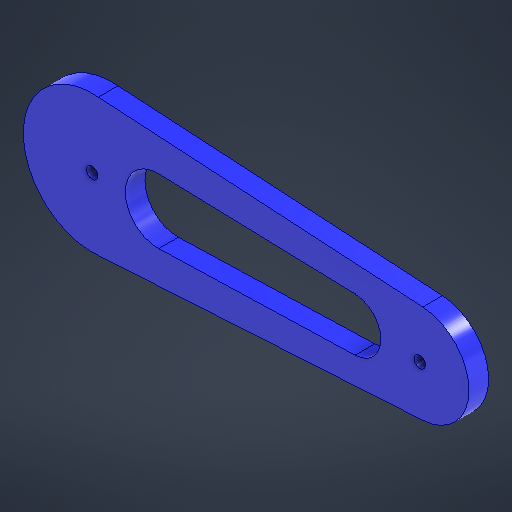
# Autodesk Inventor part: Tibia
Saved by Autodesk Inventor 2026.2 (Build 302298010, 298A)
## iProperties
Created: 2026-07-24
Part Number: Tibia
Material: Generic
Document SubType Name: Modeling
Designer: Entity
Mass: 19.7765 g
Surface Area: 96.6424 cm^2
Volume: 19.7765 cm^3
Density: 1 g/cm^3
Appearance: Blue - Wall Paint - Glossy
Author: Entity
Autodesk Inventor part; units mm, degrees
ref_plane "YZ Plane" through (0, 0, 0) normal (1, 0, 0) x (0, 1, 0)
ref_plane "XZ Plane" through (0, 0, 0) normal (0, 1, 0) x (-1, 0, 0)
ref_plane "XY Plane" through (0, 0, 0) normal (0, 0, 1) x (1, 0, 0)
sketch "Sketch1" plane through (0, 0, 0) normal (0, 0, 1) x (1, 0, 0)
  circle A0 centre (0, 0) radius 21
  circle A1 centre (100, 0) radius 15
  line L0 (0, 0) -> (100, 0)
  line L1 (0.6307, 20.9905) -> (100.8986, 14.9731)
  line L2 (0.6307, -20.9905) -> (100.8986, -14.9731)
  point P0 (100.8986, -14.9731)
  point P1 (1.8842, -20.9153)
  point P2 (1.8842, 20.9153)
  dimension "d10" = 15
  dimension "d11" = 21
  dimension "d9" = 100
  constraints: 6 end point, 2 symmetric about line, 1 coincident, 1 horizontal, 7 other
  measures "d9" distance of L0.start L0.end
extrude "Extrusion1" add sketch "Sketch1" along normal blind 6
sketch "Sketch2" plane through (0, 0, 6) normal (0, 0, 1) x (1, 0, 0)
  circle A0 centre (0, 0) radius 1.75
  arc A1 (100.8986, -14.9731) -> (100.8986, 14.9731) centre (100, 0) ccw projected
  circle A2 centre (100, 0) radius 1.75
  point P0 (293.3543, -13.4475)
  point P1 (293.3543, 13.4475)
  point P2 (250.3596, -14.9957)
  point P3 (250.3596, 14.9957)
  dimension "d5" = 3.5
  dimension "d6" = 3.5
  constraints: 2 centre point, 2 coincident, 1 other
  measures "d5" diameter of A0
  measures "d6" diameter of A2
extrude "Extrusion2" cut sketch "Sketch2" against normal through all
sketch "Sketch3" plane through (0, 0, 6) normal (0, 0, 1) x (1, 0, 0)
  circle A0 centre (0, 0) radius 1.75 projected
  line L0 (0, 0) -> (0, 10.4955)
  circle A1 centre (100, 0) radius 1.75 projected
  line L1 (100, 0) -> (100.4493, -7.4865)
  line L2 (1.8842, -20.9153) -> (100.8986, -14.9731) projected
  line L3 (0, 0) -> (100, 0)
  line L4 (0, 0) -> (0, -10.4955)
  line L5 (100, 0) -> (100.4493, 7.4865)
  line L6 (100.4493, 7.4865) -> (0, 10.4955)
  line L7 (0, -10.4955) -> (100.4493, -7.4865)
  line L8 (0, 0) -> (20, 0)
  circle A2 centre (20, 0) radius 9.892
  line L9 (100, 0) -> (80, 0)
  circle A3 centre (80, 0) radius 8.0955
  point P0 (20.1356, 12.1145)
  point P1 (20.388, 12.1119)
  point P2 (180.7309, 8.7707)
  point P3 (0.6307, -20.9905)
  point P4 (20.2962, 9.8875)
  point P5 (20.2962, -9.8875)
  point P6 (80.2424, -8.0918)
  point P7 (80.2424, 8.0918)
  dimension "d14" = 10.4955
  dimension "d15" = 7.5
  dimension "d16" = 20
  dimension "d17" = 20
  constraints: 18 end point, 2 centre point, 2 coincident, 2 point on line, 2 symmetric about line, 2 tangent, 1 horizontal, 1 perpendicular, 1 vertical
  measures "d14" distance of L0.start L0.end
  measures "d15" distance of L1.start L1.end
  measures "d16" distance of L0.start L8.end
  measures "d17" distance of L1.start L9.end
extrude "Extrusion3" cut sketch "Sketch3" against normal through all contours A2 L3 | L3 A2 | L6 A3 L3 A2 | A2 L3 A3 L7 | A3 L3 | A3 L3
body "Solid1"
